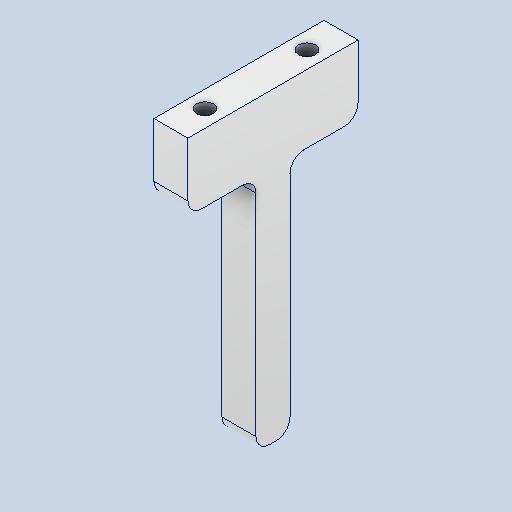
# Autodesk Inventor part: belt_liner_v1_Plate_10
Saved by Autodesk Inventor 2025.1 (Build 291241000, 241)
## iProperties
Created: 2024-12-14
Part Number: belt_liner_v1_Plate_10
Material: アルミニウム 6061
Document SubType Name: Modeling
Designer: haruy
Density: 2.7 g/cm^3
Appearance: アルミニウム - フラット
Author: haruy
Autodesk Inventor part; units mm, degrees
ref_plane "YZ Plane" through (0, 0, 0) normal (1, 0, 0) x (0, 1, 0)
ref_plane "XZ Plane" through (0, 0, 0) normal (0, 1, 0) x (-1, 0, 0)
ref_plane "XY Plane" through (0, 0, 0) normal (0, 0, 1) x (1, 0, 0)
sketch "スケッチ1" plane through (0, 0, 0) normal (1, 0, 0) x (0, 1, 0)
  line L0 (0, 0) -> (-45, 0)
  line L1 (-45, 0) -> (-45, -5)
  line L2 (-45, -5) -> (0, -5)
  line L3 (0, -5) -> (0, 0)
  line L4 (0, 10) -> (-10, 10)
  line L5 (-10, 10) -> (-10, -15)
  line L6 (-10, -15) -> (0, -15)
  line L7 (0, -15) -> (0, 10)
  point P0 (-10, 0)
  point P1 (-10, -5)
  point P2 (0, -5)
  dimension "d0" = 45
  dimension "d1" = 5
  dimension "d2" = 10
  dimension "d3" = 10
  dimension "d4" = 10
  dimension "d5" = 0
  constraints: 16 end point, 4 parallel, 2 horizontal, 2 perpendicular
  measures "d0" distance of L1.end L2.end
  measures "d1" distance of L0.end L1.end
  measures "d2" distance between parallel lines of L0 L4
  measures "d3" distance between parallel lines of L6 L2
  measures "d4" distance of L4.start L4.end
  measures "d5" distance between parallel lines of L3 L7
extrude "押し出し1" add sketch "スケッチ1" along normal blind 5
sketch "スケッチ2" plane through (0, 0, 10) normal (0, 1, 0) x (1, 0, 0)
  line L0 (0, 25) -> (5, 25) projected
  line L1 (0, 0) -> (5, 0) projected
  line L2 (0, 25) -> (0, 0) projected
  point P0 (0, 10)
  point P1 (2.5, 20)
  point P2 (2.5, 5)
  dimension "d8" = 5
  dimension "d9" = 5
  dimension "d10" = 2.5
  dimension "d11" = 2.5
  measures "d8" distance from line of L0 point (2.5, 20)
  measures "d9" distance from line of point (2.5, 5) L1
  measures "d10" distance from line of point (2.5, 5) L2
  measures "d11" distance from line of point (2.5, 20) L2
hole "穴1" at (2.5, 0, -10) at (2.5, 0, 5) direction (0, -1, 0) diameter 2.5 end through all
fillet "フィレット1" radius 2 6 edges at (2.5, -10, -15) (2.5, -10, -5) (2.5, -10, 0) (2.5, -10, 10) (2.5, -45, -5) (2.5, -45, 0)
thread "ねじ1" size "M2.5x0.45" class "6H" standard "ANSI Metric M Profile" full length
thread "ねじ2" size "M2.5x0.45" class "6H" standard "ANSI Metric M Profile" full length
